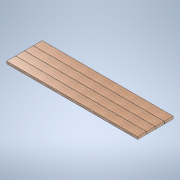
# Autodesk Inventor part: Desk Top Primary
Saved by Autodesk Inventor 2020.2 (Build 242310000, 310)
## iProperties
Created: 2019-12-30
Part Number: Desk Top Primary
Material: Wood (Birch - Stained)
Document SubType Name: Modeling
Designer: Andrew
Density: 0.1 g/cm^3
Appearance: Birch - Stained Light
l_2x4: 96.000 in
w_2x4: 3.585 in
h_2x4: 1.563 in
l_2x6: 96.000 in
w_2x6: 5.643 in
h_2x6: 1.563 in
plank_tol: 0.063 in
Author: Andrew
Autodesk Inventor part; units mm, degrees
ref_plane "YZ Plane" through (0, 0, 0) normal (1, 0, 0) x (0, 1, 0)
ref_plane "XZ Plane" through (0, 0, 0) normal (0, 1, 0) x (-1, 0, 0)
ref_plane "XY Plane" through (0, 0, 0) normal (0, 0, 1) x (1, 0, 0)
sketch "Ideal" plane through (0, 0, 0) normal (0, 1, 0) x (-1, 0, 0)
  line L0 (0, 0) -> (-2438.4, 0)
  line L1 (-2438.4, 0) -> (-2438.4, 609.6)
  line L2 (-2438.4, 609.6) -> (-609.6, 609.6)
  line L3 (-609.6, 609.6) -> (-609.6, 1219.2)
  line L4 (-609.6, 1219.2) -> (0, 1219.2)
  line L5 (0, 1219.2) -> (0, 0)
  dimension "d0" = 2438.4
  dimension "d1" = 1219.2
  dimension "d2" = 609.6
  dimension "d3" = 609.6
  dimension "d4" = 1828.8
  constraints: 12 end point, 5 perpendicular, 1 horizontal
  measures "d0" distance of L0.start L0.end
  measures "d1" distance of L4.end L0.start
  measures "d2" distance of L3.end L4.end
  measures "d3" distance of L0.end L1.end
  measures "d4" distance of L1.end L2.end
sketch "Primary Top" plane through (0, 0, 0) normal (0, 1, 0) x (-1, 0, 0)
  line L0 (-2713.228, 0) -> (-579.628, 0)
  line L1 (-579.628, 0) -> (-579.628, 143.3195)
  line L2 (-579.628, 143.3195) -> (-2713.228, 143.3195)
  line L3 (-2713.228, 143.3195) -> (-2713.228, 0)
  line L4 (-2713.228, 144.907) -> (-579.628, 144.907)
  line L5 (-579.628, 144.907) -> (-579.628, 288.2265)
  line L6 (-579.628, 288.2265) -> (-2713.228, 288.2265)
  line L7 (-2713.228, 288.2265) -> (-2713.228, 144.907)
  line L8 (-2713.228, 289.814) -> (-579.628, 289.814)
  line L9 (-579.628, 289.814) -> (-579.628, 433.1335)
  line L10 (-579.628, 433.1335) -> (-2713.228, 433.1335)
  line L11 (-2713.228, 433.1335) -> (-2713.228, 289.814)
  line L12 (-2713.228, 434.721) -> (-579.628, 434.721)
  line L13 (-579.628, 434.721) -> (-579.628, 578.0405)
  line L14 (-579.628, 578.0405) -> (-2713.228, 578.0405)
  line L15 (-2713.228, 578.0405) -> (-2713.228, 434.721)
  point P0 (0, 0)
  dimension "d5" = 143.3195
  dimension "d6" = 143.3195
  dimension "d7" = 143.3195
  dimension "d8" = 143.3195
  dimension "d9" = 2133.6
  dimension "d11" = 1.5875
  dimension "d12" = 1.5875
  dimension "d13" = 1.5875
  dimension "d17" = 579.628
  constraints: 32 end point, 8 parallel, 5 point on line, 4 horizontal, 4 perpendicular, 1 coincident, 1 collinear, 1 horizontal alignment
  measures "d5" distance of L2.end L0.start
  measures "d6" distance of L6.end L4.start
  measures "d7" distance of L10.end L8.start
  measures "d8" distance of L14.end L12.start
  measures "d9" distance of L0.start L0.end
  measures "d11" distance between parallel lines of L4 L2
  measures "d12" distance between parallel lines of L8 L6
  measures "d13" distance between parallel lines of L12 L10
  measures "d17" distance of point (0, 0) point (-579.628, 0)
extrude "Extrusion1" add sketch "Primary Top" along normal blind 39.6966
equation "\"d5\" = w_2x6"
equation "\"d6\" = d5"
equation "\"d7\" = d5"
equation "\"d8\" = d5"
equation "\"d11\" = plank_tol"
equation "\"d12\" = plank_tol"
equation "\"d13\" = plank_tol"
equation "\"d17\" = 4 * w_2x6 + 4 * plank_tol"
equation "\"d14\" = h_2x6"
equation "\"l_2x4\" = 2438.4"
equation "\"w_2x4\" = 91.059"
equation "\"h_2x4\" = 39.69657"
equation "\"l_2x6\" = 2438.4"
equation "\"w_2x6\" = 143.3195"
equation "\"h_2x6\" = h_2x4"
equation "\"plank_tol\" = 1.5875"
body "Solid1"
